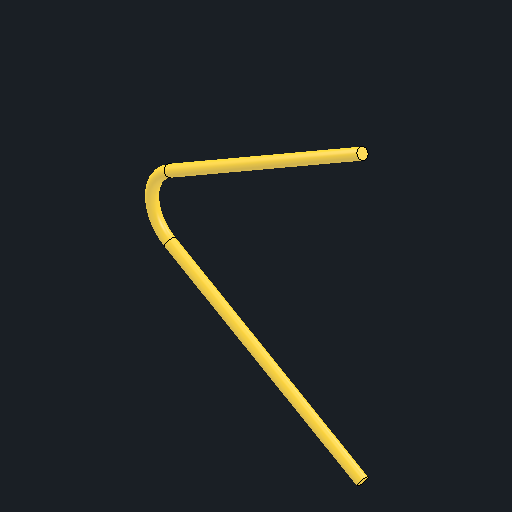
# Autodesk Inventor part: ingnition-help
Saved by Autodesk Inventor 2027.1 (Build 311270010, 270A)
## iProperties
Created: 2026-10-02
Part Number: ingnition-help
Material: Generic
Document SubType Name: Modeling
Designer: queezz
Density: 1 g/cm^3
Appearance: Glossy - Gold
Author: queezz
Autodesk Inventor part; units mm, degrees
ref_plane "YZ Plane" through (0, 0, 0) normal (1, 0, 0) x (0, 1, 0)
ref_plane "XZ Plane" through (0, 0, 0) normal (0, 1, 0) x (-1, 0, 0)
ref_plane "XY Plane" through (0, 0, 0) normal (0, 0, 1) x (1, 0, 0)
sketch "Sketch1" plane through (0, 0, 0) normal (0, 0, 1) x (1, 0, 0)
  arc A0 (-0.875, 1.5155) -> (-0.875, -1.5155) centre (0, 0) ccw
  line L0 (-0.875, 1.5155) -> (8.6513, 7.0155)
  line L1 (-0.875, -1.5155) -> (8.6513, -7.0155)
  dimension "d0" = 3.5
  dimension "d1" = 11
  dimension "d2" = 60
  constraints: 4 end point, 2 point on circle, 2 tangent, 2 vertical alignment, 1 centre point, 1 coincident
  measures "d0" diameter of A0
  measures "d1" distance of L0.start L0.end
  measures "d2" angle of L1 L0
sketch "Sketch2" plane through (0, 0, 0) normal (0, 1, 0) x (-1, 0, 0)
  circle A0 centre (1.75, 0) radius 0.25
  line L0 (1.75, 0) -> (0.875, 0) projected
  point P0 (0, 0)
  point P1 (0.875, 0)
  dimension "d3" = 0.5
  constraints: 1 centre point, 1 coincident
  measures "d3" diameter of A0
sweep "Sweep1" add profiles "Sketch2" path "Sketch1"
body "Solid1"
